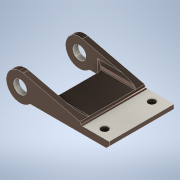
# Autodesk Inventor part: Part13 Half Hinge
Saved by Autodesk Inventor 2022.2 (Build 262287010, 287A)
## iProperties
Created: 2022-12-08
Part Number: Part13 Half Hinge
Material: Steel, Carbon
Document SubType Name: Modeling
Designer: User
Density: 7.85 g/cm^3
Appearance: Gunmetal - Antique Polished
Mass: 126.663 g
Surface Area: 78.4583 cm^2
Volume: 16.1354 cm^3
Author: User
Autodesk Inventor part; units mm, degrees
ref_plane "YZ Plane" through (0, 0, 0) normal (1, 0, 0) x (0, 1, 0)
ref_plane "XZ Plane" through (0, 0, 0) normal (0, 1, 0) x (-1, 0, 0)
ref_plane "XY Plane" through (0, 0, 0) normal (0, 0, 1) x (1, 0, 0)
sketch "Sketch1" plane through (0, 0, 0) normal (0, 0, 1) x (1, 0, 0)
  arc A0 (2.3256, 9.7258) -> (7.1414, -7) centre (0, 0) ccw
  line L0 (7.1414, -7) -> (64, -7)
  line L1 (64, -7) -> (64, -2)
  line L2 (64, -2) -> (45, -2)
  arc A1 (43, 0) -> (45, -2) centre (45, 0) ccw
  line L3 (43, 0) -> (2.3256, 9.7258)
  dimension "d0" = 10
  dimension "d1" = 2
  dimension "d2" = 5
  dimension "d3" = 64
  dimension "d4" = 21
  constraints: 8 end point, 4 point on circle, 2 centre point, 2 horizontal alignment, 2 perpendicular, 2 tangent, 1 coincident, 1 horizontal
  measures "d0" radius of A0
  measures "d1" radius of A1
  measures "d2" distance between parallel lines of L0 L2
  measures "d3" distance from line of A0.centre L1
  measures "d4" distance from line of L3.start L1
extrude "Extrusion1" add sketch "Sketch1" along normal mid plane 46.5
sketch "Sketch2" plane through (64, -7, 23.25) normal (1, 0, 0) x (0, 0, -1)
  line L0 (0, 16.7258) -> (46.5, 16.7258) construction
  line L1 (3.85, 17) -> (42.65, 17)
  line L2 (42.65, 17) -> (42.65, 10)
  line L3 (39.65, 7) -> (6.85, 7)
  line L4 (3.85, 10) -> (3.85, 17)
  line L5 (46.5, 17) -> (0, 17) construction
  arc A0 (3.85, 10) -> (6.85, 7) centre (6.85, 10) ccw
  arc A1 (39.65, 7) -> (42.65, 10) centre (39.65, 10) ccw
  point P0 (23.25, 7)
  point P1 (23.25, 7)
  dimension "d7" = 38.8
  dimension "d8" = 3
  constraints: 8 end point, 4 point on circle, 4 tangent, 2 centre point, 2 parallel, 1 coincident, 1 collinear, 1 equal radius, 1 horizontal, 1 midpoint, 1 perpendicular
  measures "d7" distance of L1.start L1.end
  measures "d8" radius of A0
extrude "Extrusion2" cut sketch "Sketch2" against normal through all
sketch "Sketch3" plane through (-10, 0, 16.4) normal (0, 1, 0) x (1, 0, 0)
  line L0 (0, 0) -> (0, 32.8) construction
  line L1 (12.3256, 35.8) -> (0.4606, 35.8) construction
  line L2 (0.4606, -3) -> (12.3256, -3) construction
  line L3 (0, 35.8) -> (23, 35.8)
  line L4 (29, 29.8) -> (29, 3)
  line L5 (23, -3) -> (0, -3)
  line L6 (0, -3) -> (0, 35.8)
  line L7 (40.4537, 35.8) -> (0.4606, 35.8) projected
  line L8 (40.4537, -3) -> (0.4606, -3) projected
  arc A0 (29, 29.8) -> (23, 35.8) centre (23, 29.8) ccw
  arc A1 (23, -3) -> (29, 3) centre (23, 3) ccw
  arc A2 (29, 29.8) -> (23, 35.8) centre (23, 29.8) ccw
  arc A3 (23, -3) -> (29, 3) centre (23, 3) ccw
  point P0 (10, 16.4)
  dimension "d11" = 29
  dimension "d12" = 6
  constraints: 8 end point, 8 point on circle, 8 tangent, 4 centre point, 4 point on line, 3 collinear, 3 equal radius, 2 parallel, 1 horizontal, 1 perpendicular
  measures "d11" distance between parallel lines of L4 L0
  measures "d12" radius of A0
extrude "Extrusion3" cut sketch "Sketch3" along normal through all both and the other way through all
fillet "Fillet1" radius 2 2 edges at (7.1414, -7, 21.325) (7.1414, -7, -21.325)
chamfer "Chamfer1" distance 2 angle 45 1 edges at (64, -7, 0)
sketch "Sketch4" plane through (0, 0, 23.25) normal (0, 0, 1) x (1, 0, 0)
  arc A0 (2.3256, 9.7258) -> (6.6144, -7.5) centre (0, 0) ccw projected
  constraints: 1 coincident
hole "Hole1" at (0, 0, 23.25) direction (0, 0, -1) diameter 9.5 end through all
sketch "Sketch5" plane through (45, -2, 23.25) normal (0, 1, 0) x (1, 0, 0)
  line L0 (19, 0) -> (0, 0) projected
  line L1 (19, 46.5) -> (19, 0) projected
  line L2 (0, 46.5) -> (19, 46.5) projected
  point P0 (-45, 23.25)
  point P1 (9.5, 40.25)
  point P2 (9.5, 6.25)
  dimension "d26" = 34
  dimension "d27" = 6.25
  dimension "d28" = 6.25
  dimension "d29" = 9.5
  measures "d26" distance of point (9.5, 6.25) point (9.5, 40.25)
  measures "d27" distance from line of point (9.5, 40.25) L2
  measures "d28" distance from line of point (9.5, 6.25) L0
  measures "d29" distance from line of L1 point (9.5, 40.25)
hole "Hole2" at (54.5, -2, -17) at (54.5, -2, 17) direction (0, -1, 0) diameter 5.2 end through all
body "Solid1"
